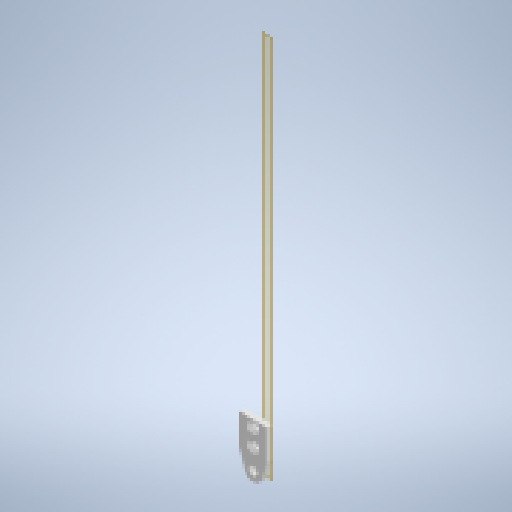
# Autodesk Inventor part: belt_tentioner_2
Saved by Autodesk Inventor 2024 (Build 280153000, 153)
## iProperties
Created: 2026-02-16
Part Number: belt_tentioner_2
Material: Generic
Document SubType Name: Modeling
Designer: SEMEN
Density: 1 g/cm^3
Appearance: Default
Author: SEMEN
Autodesk Inventor part; units mm, degrees
ref_plane "YZ Plane" through (0, 0, 0) normal (1, 0, 0) x (0, 1, 0)
ref_plane "XZ Plane" through (0, 0, 0) normal (0, 1, 0) x (-1, 0, 0)
ref_plane "XY Plane" through (0, 0, 0) normal (0, 0, 1) x (1, 0, 0)
ref_plane "Work Plane1" through (0, 0, 0) normal (0, 0, 1) x (1, 0, 0)
sketch "Sketch1" plane through (0, 0, 0) normal (0, 0, 1) x (1, 0, 0)
  circle A0 centre (-3, 740) radius 5.2 projected
  circle A1 centre (-3, 767) radius 4.3 projected
  circle A2 centre (-3, 755) radius 4.3 projected
  line L0 (7, 772) -> (7, 750) projected
  line L1 (7, 750) -> (3.1945, 738.0305) projected
  arc A3 (-9.1945, 738.0305) -> (3.1945, 738.0305) centre (-3, 740) ccw projected
  line L2 (-9.1945, 738.0305) -> (-13, 750) projected
  line L3 (-13, 750) -> (-13, 772) projected
  line L4 (-13, 772) -> (7, 772) projected
  point P0 (0, 0)
extrude "Extrusion1" add sketch "Sketch1" along normal blind 4 contours A0 | A1 | A2 | L0 L1 A3 L2 L3 L4
hole "Hole1" at (-3, 740, 0) direction (0, 0, 1) diameter 5.5 end through all clearance for "Countersunk Head GOST 12876-67" size "M5" standard "GOST"
sketch "Sketch2" plane through (0, 0, 4) normal (0, 0, 1) x (1, 0, 0)
  circle A0 centre (-3, 740) radius 5.2 projected
  circle A1 centre (-3, 767) radius 4.3 projected
  circle A2 centre (-3, 755) radius 4.3 projected
  line L0 (7, 772) -> (7, 750) projected
  line L1 (7, 750) -> (3.1945, 738.0305) projected
  arc A3 (-9.1945, 738.0305) -> (3.1945, 738.0305) centre (-3, 740) ccw projected
  line L2 (-9.1945, 738.0305) -> (-13, 750) projected
  line L3 (-13, 750) -> (-13, 772) projected
  line L4 (-13, 772) -> (7, 772) projected
  point P0 (0, 0)
hole "Hole2" at (-3, 767, 4) at (-3, 755, 4) direction (0, 0, -1) diameter 4.5 end through all countersink diameter 8.6 countersink angle 90 clearance for "Countersunk Head GOST 12876-67" size "M4" standard "GOST"
body "Solid1"
